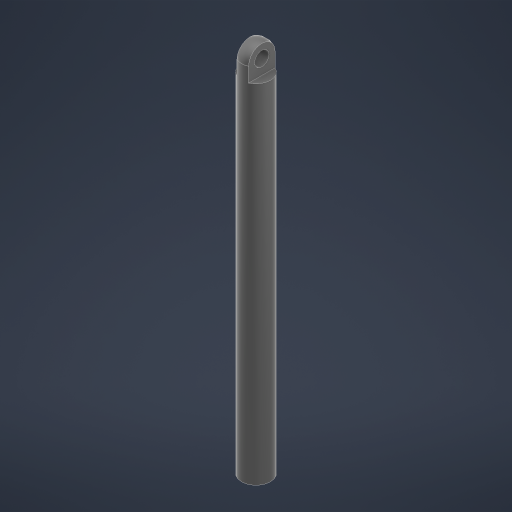
# Autodesk Inventor part: FP V2 Shaft
Saved by Autodesk Inventor 2023.6 (Build 276521000, 521)
## iProperties
Created: 2026-02-12
Part Number: FP V2 Shaft
Material: Aluminum 6061
Document SubType Name: Modeling
Designer: user
Density: 2.7 g/cm^3
Appearance: Smooth - Black
Author: user
Autodesk Inventor part; units mm, degrees
ref_plane "YZ Plane" through (0, 0, 0) normal (1, 0, 0) x (0, 1, 0)
ref_plane "XZ Plane" through (0, 0, 0) normal (0, 1, 0) x (-1, 0, 0)
ref_plane "XY Plane" through (0, 0, 0) normal (0, 0, 1) x (1, 0, 0)
sketch "Sketch1" plane through (0, 0, 0) normal (0, 1, 0) x (-1, 0, 0)
  circle A0 centre (0, 0) radius 5
  dimension "d0" = 10
  constraints: 1 centre point, 1 coincident
  measures "d0" diameter of A0
extrude "Extrusion1" add sketch "Sketch1" along normal blind 120
sketch "Sketch3" plane through (0, 120, 0) normal (0, 1, 0) x (1, 0, 0)
  circle A0 centre (0, 0) radius 5 projected
  line L0 (0, 0) -> (0, 9.0773)
  line L1 (-5, 0) -> (-2, 0)
  line L2 (-2, 0) -> (-2, 4.5826)
  line L3 (-2, 0) -> (-2, -4.5826)
  line L4 (5, 0) -> (2, 0)
  line L5 (2, 0) -> (2, 4.5826)
  line L6 (2, 0) -> (2, -4.5826)
  dimension "d7" = 3
  dimension "d8" = 3
  constraints: 14 end point, 6 point on circle, 4 point on line, 2 perpendicular, 1 horizontal, 1 vertical
  measures "d7" distance of L1.start L1.end
  measures "d8" distance of L4.start L4.end
extrude "Extrusion3" add sketch "Sketch3" along normal blind 10 contours L5 L6 A0 L3 L2
sketch "Sketch4" plane through (-2, 120, -4.5826) normal (-1, 0, 0) x (0, 0, 1)
  line L0 (9.1652, 0) -> (0, 0) projected
  line L1 (9.1652, 0) -> (9.1652, 10) projected
  line L2 (0, 10) -> (9.1652, 10) projected
  line L3 (0, 0) -> (0, 10) projected
  line L4 (0, 0) -> (9.1652, 0) projected
  line L5 (0, 0) -> (0, 10) projected
  line L6 (9.1652, 10) -> (0, 10) projected
  line L7 (9.1652, 0) -> (9.1652, 10) projected
  line L8 (9.1652, 0) -> (0, 0) projected
  line L9 (4.5826, 0) -> (4.5826, 5)
  circle A0 centre (4.5826, 5) radius 2.5
  point P0 (4.5826, -120)
  dimension "d11" = 5
  constraints: 2 end point, 1 centre point, 1 coincident, 1 midpoint, 1 vertical
  measures "d11" diameter of A0
extrude "Extrusion4" cut sketch "Sketch4" against normal blind 10 contours A0
fillet "Fillet1" radius 5 1 edges at (0, 130, 5)
body "Solid1"
